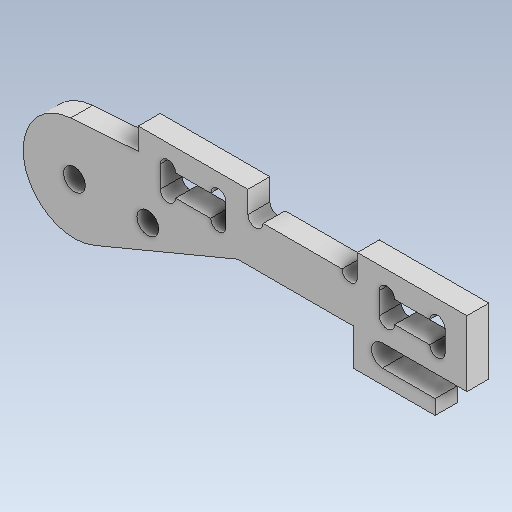
# Autodesk Inventor part: シールド先端接続
Saved by Autodesk Inventor 2020 (Build 240168000, 168)
## iProperties
Created: 2020-02-10
Part Number: シールド先端接続
Material: 一般
Document SubType Name: Modeling
Designer: tanjihayato
Density: 1 g/cm^3
Appearance: 既定
Mass: 1.60794 g
Surface Area: 18.3491 cm^2
Volume: 1.60794 cm^3
Author: tanjihayato
Autodesk Inventor part; units mm, degrees
ref_plane "YZ Plane" through (0, 0, 0) normal (1, 0, 0) x (0, 1, 0)
ref_plane "XZ Plane" through (0, 0, 0) normal (0, 1, 0) x (-1, 0, 0)
ref_plane "XY Plane" through (0, 0, 0) normal (0, 0, 1) x (1, 0, 0)
sketch "スケッチ1" plane through (0, 0, 0) normal (0, 0, 1) x (1, 0, 0)
  line L0 (0, 0) -> (0, -3)
  line L1 (0, 0) -> (-15, 0)
  line L2 (-15, 0) -> (-15, -3)
  line L3 (-15, -3) -> (-30, -3)
  line L4 (-30, -3) -> (-30, 0)
  line L5 (-30, 0) -> (-45, 0)
  line L6 (-45, 0) -> (-45, -3)
  line L7 (-257.4775, 0) -> (-66.4062, 0)
  line L8 (-66.4062, 0) -> (-51.9242, -3.906)
  line L9 (-257.4775, 0) -> (-257.4775, -3)
  line L10 (-257.4775, -3) -> (-68.9626, -6)
  line L11 (-68.9626, -6) -> (-58.5737, -15.799)
  circle A0 centre (-53.7535, -10.6886) radius 4.025
  circle A1 centre (-53.7535, -10.6886) radius 1.5
  line L12 (0, -3) -> (0, -9)
  arc A2 (-54.2694, -3.6826) -> (-51.0532, -17.1739) centre (-53.7535, -10.6886) ccw
  line L13 (-54.2694, -3.6826) -> (-45, -3)
  line L14 (-51.0532, -17.1739) -> (-31.4218, -9)
  line L15 (-31.4218, -9) -> (0, -9)
  arc A3 (-46.7293, -10.7926) -> (-42.5418, -13.63) centre (-43.7046, -10.8374) ccw
  circle A4 centre (-43.7046, -10.8374) radius 1.5
  line L16 (-54.6828, -17.6519) -> (-41.7856, -19.3732)
  arc A5 (-41.7856, -19.3732) -> (-42.5418, -13.63) centre (-41.3887, -16.3996) ccw
  arc A6 (-58.5737, -15.799) -> (-54.6828, -17.6519) centre (-53.7535, -10.6886) ccw
  arc A7 (-46.7293, -10.7926) -> (-51.9242, -3.906) centre (-53.7535, -10.6886) ccw
  line L17 (-42, -3) -> (-33, -3)
  line L18 (-33, -3) -> (-33, -6)
  line L19 (-33, -6) -> (-42, -6)
  line L20 (-42, -6) -> (-42, -3)
  line L21 (-12, -3) -> (-3, -3)
  line L22 (-3, -3) -> (-3, -6)
  line L23 (-3, -6) -> (-12, -6)
  line L24 (-12, -6) -> (-12, -3)
  circle A8 centre (-40.95, -3) radius 1.05
  circle A9 centre (-34.05, -3) radius 1.05
  circle A10 centre (-34.05, -6) radius 1.05
  circle A11 centre (-40.95, -6) radius 1.05
  circle A12 centre (-10.95, -3) radius 1.05
  circle A13 centre (-4.05, -3) radius 1.05
  circle A14 centre (-4.05, -6) radius 1.05
  circle A15 centre (-10.95, -6) radius 1.05
  circle A16 centre (-28.95, -3) radius 1.05
  circle A17 centre (-16.05, -3) radius 1.05
  circle A18 centre (-41.3887, -16.3996) radius 1.25
  line L25 (-15.5802, -9) -> (-15.5802, -14)
  line L26 (-15.5802, -14) -> (-4.3492, -14)
  line L27 (-4.3492, -14) -> (-4.3492, -12)
  line L28 (-4.3492, -12) -> (-11.5802, -12)
  arc A19 (-11.5802, -9) -> (-11.5802, -12) centre (-11.5802, -10.5) ccw
  point P0 (-5.1, -6)
  point P1 (-9.9, -6)
  point P2 (-9.9, -3)
  point P3 (-5.1, -3)
  point P4 (-35.1, -6)
  point P5 (-39.9, -6)
  point P6 (-39.9, -3)
  point P7 (-35.1, -3)
  point P8 (-17.1, -3)
  point P9 (-27.9, -3)
  dimension "d0" = 3
  dimension "d1" = 15
  dimension "d2" = 3
  dimension "d3" = 15
  dimension "d5" = 15
  dimension "d6" = 3
  dimension "d7" = 3
  dimension "d8" = 8.05
  dimension "d10" = 3
  dimension "d11" = 6
  dimension "d12" = 6
  dimension "d13" = 6.05
  dimension "d14" = 3
  dimension "d15" = 9
  dimension "d16" = 3
  dimension "d17" = 9
  dimension "d18" = 3
  dimension "d19" = 3
  dimension "d20" = 3
  dimension "d21" = 3
  dimension "d22" = 3
  dimension "d23" = 3
  dimension "d24" = 2.1
  dimension "d25" = 2.1
  dimension "d26" = 2.1
  dimension "d27" = 2.1
  dimension "d28" = 2.1
  dimension "d29" = 2.1
  dimension "d30" = 2.1
  dimension "d31" = 2.1
  dimension "d32" = 2.1
  dimension "d33" = 2.1
  dimension "d34" = 2.5
  dimension "d36" = 3
  dimension "d37" = 3
  dimension "d38" = 2
  dimension "d39" = 4
  constraints: 58 end point, 22 tangent, 20 centre point, 16 point on line, 12 point on circle, 7 perpendicular, 6 vertical, 5 coincident, 5 horizontal, 4 parallel, 2 collinear
  measures "d0" distance of L0.start L0.end
  measures "d1" distance of L0.start L1.end
  measures "d2" distance of L1.end L2.end
  measures "d3" distance of L2.end L3.end
  measures "d5" distance of L4.end L5.end
  measures "d6" distance of L5.end L6.end
  measures "d7" distance of L7.start L9.end
  measures "d8" diameter of A0
  measures "d10" diameter of A1
  measures "d11" distance of L0.end L12.end
  measures "d12" distance from line of L7 L10.end
  measures "d13" diameter of A3
  measures "d14" diameter of A4
  measures "d15" distance of L18.end L19.end
  measures "d16" distance of L17.end L18.end
  measures "d17" distance of L22.end L23.end
  measures "d18" distance of L21.end L22.end
  measures "d19" radial gap between concentric circles of A2 A0
  measures "d20" radial gap between concentric circles of A6 A0
  measures "d21" radial gap between concentric circles of A7 A0
  measures "d22" distance between parallel lines of L18 L4
  measures "d23" distance between parallel lines of L24 L2
  measures "d24" diameter of A8
  measures "d25" diameter of A9
  measures "d26" diameter of A10
  measures "d27" diameter of A11
  measures "d28" diameter of A12
  measures "d29" diameter of A13
  measures "d30" diameter of A14
  measures "d31" diameter of A15
  measures "d32" diameter of A16
  measures "d33" diameter of A17
  measures "d34" diameter of A18
  measures "d36" radius of A5
  measures "d37" distance between parallel lines of L28 L15
  measures "d38" distance between parallel lines of L26 L28
  measures "d39" distance from line of L25 A19.centre
extrude "押し出し1" add sketch "スケッチ1" along normal blind 3 contours L0 L12 L15 L14 A3 A7 L8 L13 L6 L5 L4 A16 L3 A17 L2 L1 | A19 L28 L27 L26 L25 L15 | L14 A2 L13 L8 A7 A3 | A0
